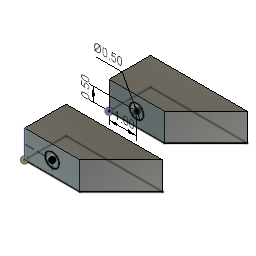
3.1_Example (Autodesk Fusion 360 design; units mm, degrees)
Autodesk Fusion 360 part; units mm, degrees
sketch "Sketch1" plane through (0, 0, 0) normal (0, 0, 1) x (1, 0, 0)
  line L0 (0, 0) -> (50.8, 0)
  line L1 (50.8, 0) -> (88.9, 38.1)
  line L2 (88.9, 38.1) -> (0, 38.1)
  line L3 (0, 38.1) -> (0, 0)
  line L4 (-0.0164, -77.6551) -> (50.7836, -77.6551)
  line L5 (50.7836, -77.6551) -> (88.8781, -39.5935)
  line L6 (88.8781, -39.5935) -> (0, -39.5551)
  line L7 (-0.0164, -77.6551) -> (0, -39.5551)
  dimension "d1" = 50.8
  dimension "d2" = 38.1
  dimension "d3" = 45
  dimension "d4" = 50.8
  dimension "d5" = 38.1
  dimension "d6" = 45
  constraint coincident L0.start L3.end
  constraint horizontal L0
  constraint perpendicular L0 L3
  constraint vertical L0.start L6.end
  constraint perpendicular L2 L3
  constraint horizontal L4
  constraint perpendicular L6 L7
  measures "d1" distance of L0.start L0.end
  measures "d2" distance of L2.end L0.start
  measures "d3" angle of L1 L2
  measures "d4" distance of L4.end L4.start
  measures "d5" distance of L6.end L4.start
  measures "d6" angle of L5 L6
extrude "Extrude1" add sketch "Sketch1" along normal blind 25.4 makes body 1 at (46.5667, 25.4, 0) makes body 2 at (46.5539, -52.2679, 0)
sketch "Sketch2" plane through (0, 0, 0) normal (0, -1, 0) x (1, 0, 0)
  line L0 (0, 0) -> (50.8, 0)
  line L1 (50.8, 0) -> (50.8, 25.4)
  line L2 (50.8, 25.4) -> (0, 25.4)
  line L3 (0, 25.4) -> (0, 0)
  circle A0 centre (25.4, 12.7) radius 6.35
  dimension "d9" = 12.7
  dimension "d10" = 25.4
  dimension "d11" = 12.7
  measures "d9" vertical distance of L0.start A0.centre
  measures "d10" horizontal distance of L0.start A0.centre
  measures "d11" diameter of A0
sketch "Sketch3" plane through (0, -77.6551, 0) normal (0, -1, 0) x (1, 0, 0)
  line L0 (-0.0164, 0) -> (50.7836, 0)
  line L1 (50.7836, 0) -> (50.7836, 25.4)
  line L2 (50.7836, 25.4) -> (-0.0164, 25.4)
  circle A0 centre (25.3836, 12.7) radius 6.35
  line L3 (-0.0164, 12.7) -> (25.3836, 12.7) construction
  line L4 (25.3836, 12.7) -> (25.3836, 0) construction
  line L5 (-0.0164, 25.4) -> (-0.0164, 0)
  dimension "d12" = 12.7
  constraint coincident A0.centre L3.end
  constraint midpoint L0 L4.end
  constraint horizontal L3
  constraint vertical L4
  constraint midpoint L3.start L5
  measures "d12" diameter of A0
extrude "Extrude2" cut sketch "Sketch2" against normal blind 25.4 contours A0 bodies 1
extrude "Extrude3" cut sketch "Sketch3" against normal through all contours A0 bodies 2
named bodies: "Example 01", "Example 02"
